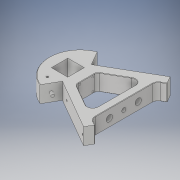
# Autodesk Inventor part: Profil_Winkel_oben
Saved by Autodesk Inventor 2019 (Build 230136000, 136)
## iProperties
Created: 2018-08-17
Part Number: Profil_Winkel_oben
Material: Generic
Document SubType Name: Modeling
Designer: Julia
Density: 1 g/cm^3
Appearance: Default
Author: Julia
Autodesk Inventor part; units mm, degrees
ref_plane "YZ Plane" through (0, 0, 0) normal (1, 0, 0) x (0, 1, 0)
ref_plane "XZ Plane" through (0, 0, 0) normal (0, 1, 0) x (-1, 0, 0)
ref_plane "XY Plane" through (0, 0, 0) normal (0, 0, 1) x (1, 0, 0)
sketch "Sketch1" plane through (0, 0, 0) normal (0, 1, 0) x (-1, 0, 0)
  line L0 (-126.3701, 48.161) -> (-51.2671, 4.8003) construction
  line L1 (-51.2671, 4.8003) -> (-126.3701, -38.5605) construction
  line L2 (-126.3701, -38.5605) -> (-126.3701, 48.161) construction
  line L3 (110.9585, 0) -> (-59.5814, 0) construction
  line L4 (83.2089, 69.641) -> (63.2089, 35)
  line L5 (63.2089, 35) -> (-58.0347, 105)
  line L6 (-58.0347, 105) -> (-68.0347, 87.6795)
  line L7 (-68.0347, 87.6795) -> (-50.7142, 77.6795)
  line L8 (-33.3937, 67.6795) -> (40.2185, 25.1795)
  line L9 (83.2089, -69.641) -> (63.2089, -35)
  line L10 (63.2089, -35) -> (-58.0347, -105)
  line L11 (-58.0347, -105) -> (-68.0347, -87.6795)
  line L12 (-68.0347, -87.6795) -> (-50.7142, -77.6795)
  line L13 (-33.3937, -67.6795) -> (40.2185, -25.1795)
  arc A0 (83.2089, -69.641) -> (83.2089, 69.641) centre (55.3678, 0) ccw
  line L14 (-50.7142, 77.6795) -> (-50.7142, -77.6795)
  line L15 (-33.3937, 67.6795) -> (-33.3937, -67.6795)
  line L16 (40.2185, 25.1795) -> (40.2185, -25.1795)
  dimension "d3" = 40
  dimension "d4" = 140
  dimension "d5" = 20
  dimension "d7" = 20
  dimension "d19" = 70
  dimension "d20" = 75
  dimension "d21" = 20
  dimension "d22" = 85
  constraints: 34 end point, 7 symmetric about line, 5 vertical, 4 perpendicular, 2 equal length, 2 horizontal, 2 point on circle, 1 centre point, 1 collinear, 1 parallel, 1 point on line, 3 other
  measures "d3" distance of L4.start L4.end
  measures "d4" distance of L4.end L5.end
  measures "d5" distance of L5.end L6.end
  measures "d7" distance of L6.end L7.end
  measures "d19" distance of L9.end L4.end
  measures "d20" radius of A0
  measures "d21" distance of L8.start L7.end
  measures "d22" distance of L8.start L8.end
extrude "Extrusion1" add sketch "Sketch1" along normal blind 40
sketch "Sketch2" plane through (-63.2089, 0, 35) normal (0.8660254, 0, 0.5) x (0.5, 0, -0.8660254)
  circle A0 centre (-20, 20) radius 3.4
  line L0 (-40, 40) -> (0, 40) projected
  line L1 (-40, 0) -> (-40, 40) projected
  point P0 (61.9153, 0)
  point P1 (-20, 40)
  point P2 (-40, 20)
  dimension "d10" = 6.8
  constraints: 2 midpoint, 1 centre point, 1 horizontal alignment, 1 vertical alignment
  measures "d10" diameter of A0
extrude "Extrusion2" add sketch "Sketch2" along normal blind 10
sketch "Sketch3" plane through (-83.2089, 0, -69.641) normal (0.8660254, 0, -0.5) x (-0.5, 0, -0.8660254)
  circle A0 centre (-20, 20) radius 3.4
  line L0 (-40, 40) -> (0, 40) projected
  line L1 (0, 0) -> (0, 40) projected
  point P0 (-101.9153, 0)
  point P1 (-20, 40)
  point P2 (0, 20)
  dimension "d13" = 6.8
  constraints: 2 midpoint, 1 centre point, 1 horizontal alignment, 1 vertical alignment
  measures "d13" diameter of A0
extrude "Extrusion3" add sketch "Sketch3" along normal blind 10
sketch "Sketch4" plane through (0, 40, 0) normal (0, 1, 0) x (1, 0, 0)
  line L0 (-105.2185, -20) -> (-65.2185, -20)
  line L1 (-65.2185, -20) -> (-65.2185, 20)
  line L2 (-65.2185, 20) -> (-105.2185, 20)
  line L3 (-105.2185, 20) -> (-105.2185, -20)
  line L4 (-40.2185, -25.1795) -> (-40.2185, 25.1795) projected
  point P0 (0, 0)
  point P1 (-105.2185, 0)
  dimension "d16" = 40
  dimension "d17" = 40
  dimension "d23" = 25
  constraints: 8 end point, 2 parallel, 1 horizontal, 1 horizontal alignment, 1 midpoint, 1 perpendicular
  measures "d16" distance of L2.end L0.start
  measures "d17" distance of L1.end L2.end
  measures "d23" distance between parallel lines of L1 L4
extrude "Extrusion4" cut sketch "Sketch4" against normal blind 40
fillet "Fillet1" radius 10 2 edges at (-40.2185, 20, -25.1795) (-40.2185, 20, 25.1795)
fillet "Fillet2" radius 13 2 edges at (33.3937, 20, 67.6795) (33.3937, 20, -67.6795)
fillet "Fillet3" radius 15 2 edges at (50.7142, 20, 77.6795) (50.7142, 20, -77.6795)
sketch "Sketch5" plane through (68.0347, 0, 87.6795) normal (0.5, 0, -0.8660254) x (-0.8660254, 0, -0.5)
  point P0 (102.7595, 0)
  point P1 (5.815, 19.918)
hole "Hole1" at (62.9988, 19.918, 84.772) direction (-0.5, 0, 0.8660254) diameter 4 end through all counterbore diameter 5 counterbore depth 2
sketch "Sketch6" plane through (-35.2185, 0, 28.0662) normal (0.5, 0, -0.8660254) x (-0.8660254, 0, -0.5)
  point P0 (-16.467, 0)
  point P1 (-7.7378, 18.9937)
hole "Hole2" at (-28.5174, 18.9937, 31.9351) direction (-0.5, 0, 0.8660254) diameter 4 end through all counterbore diameter 5 counterbore depth 2
fillet "Fillet8" radius 1 28 edges at (-38.8788, 0, 24.406) (-10.6624, 0, 42.2437) (26.8937, 0, 56.4212) (33.3937, 0, 0) (26.8937, 0, -56.4212) (-10.6624, 0, -42.2437) (-38.8788, 0, -24.406) (-40.2185, 0, 0) (52.7238, 0, -76.5192) (63.1244, 0, -84.8446) (52.7238, 0, 76.5192) (63.1244, 0, 84.8446) (50.7142, 0, 0) (-38.8788, 40, -24.406) (-10.6624, 40, -42.2437) (26.8937, 40, -56.4212) (33.3937, 40, 0) (26.8937, 40, 56.4212) (-10.6624, 40, 42.2437) (-38.8788, 40, 24.406) (-40.2185, 40, 0) (52.7238, 40, -76.5192) (63.1244, 40, -84.8446) (52.7238, 40, 76.5192) (63.1244, 40, 84.8446) (50.7142, 40, 0) (68.0347, 20, 87.6795) (68.0347, 20, -87.6795)
fillet "Fillet9" radius 1 2 edges at (-130.3678, 0, 0) (-130.3678, 40, 0)
sketch "Sketch7" plane through (0, 40, 0) normal (0, 1, 0) x (1, 0, 0)
  point P0 (0, 0)
  point P1 (-90.7612, -44.0721)
hole "Hole3" at (-90.7612, 40, 44.0721) direction (0, -1, 0) diameter 4 end through all counterbore diameter 5 counterbore depth 2
sketch "Sketch8" plane through (50.7142, 1, 69.0192) normal (1, 0, 0) x (0, 0, -1)
  circle A0 centre (34.0192, 18) radius 7.5
  circle A1 centre (104.0192, 18) radius 7.5
  line L0 (97.0855, 0) -> (97.0855, 38) projected
  line L1 (0, 38) -> (138.0385, 38) projected
  circle A2 centre (69.0192, 18) radius 5
  point P0 (69.0192, -1)
  dimension "d56" = 15
  dimension "d57" = 15
  dimension "d58" = 20
  dimension "d59" = 35
  dimension "d60" = 35
  dimension "d82" = 10
  constraints: 3 centre point, 2 horizontal alignment, 1 vertical alignment
  measures "d56" diameter of A0
  measures "d57" diameter of A1
  measures "d58" distance from line of L1 A0.centre
  measures "d59" horizontal distance of A1.centre point (69.019, -1)
  measures "d60" horizontal distance of A0.centre point (69.019, -1)
  measures "d82" diameter of A2
sketch "Sketch9" plane through (-40.2185, 1, 19.406) normal (1, 0, 0) x (0, 0, -1)
  line L0 (0, 38) -> (38.812, 38) projected
  line L1 (19.406, 38) -> (19.406, 0) construction
  line L2 (38.812, 0) -> (0, 0) projected
  line L3 (0, 19) -> (38.812, 19) construction
  line L4 (0, 0) -> (0, 38) projected
  line L5 (38.812, 38) -> (38.812, 0) projected
  point P0 (19.406, -1)
  point P1 (3.906, 34.5)
  point P2 (34.906, 34.5)
  point P3 (3.906, 3.5)
  point P4 (34.906, 3.5)
  dimension "d64" = 19
  dimension "d67" = 15.5
  dimension "d68" = 15.5
  dimension "d69" = 15.5
  dimension "d70" = 15.5
  dimension "d71" = 15.5
  dimension "d72" = 15.5
  dimension "d73" = 15.5
  dimension "d74" = 15.5
  constraints: 4 end point, 4 midpoint, 1 horizontal
  measures "d64" distance between parallel lines of L3 L0
  measures "d67" distance from line of L1 point (3.906, 34.5)
  measures "d68" distance from line of L3 point (3.906, 34.5)
  measures "d69" distance from line of L3 point (34.906, 34.5)
  measures "d70" distance from line of point (34.906, 34.5) L1
  measures "d71" distance from line of point (3.906, 3.5) L1
  measures "d72" distance from line of point (3.906, 3.5) L3
  measures "d73" distance from line of L3 point (34.906, 3.5)
  measures "d74" distance from line of point (34.906, 3.5) L1
hole "Hole4" at (-40.2185, 35.5, 15.5) at (-40.2185, 35.5, -15.5) at (-40.2185, 4.5, 15.5) at (-40.2185, 4.5, -15.5) direction (-1, 0, 0) diameter 4 depth 15 tip angle 118
extrude "Extrusion6" cut sketch "Sketch8" against normal blind 20
body "Solid1"
